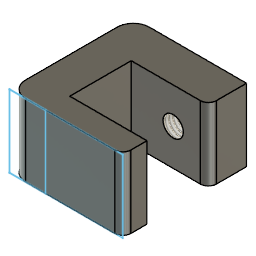
deck2plateClamp_I1 (Autodesk Fusion 360 design; units mm, degrees)
part number: 2026-05-03-05-26-52-082
Autodesk Fusion 360 part; units mm, degrees
sketch "Sketch1" plane through (0, 0, 0) normal (0, 1, 0) x (1, 0, 0)
  line L0 (-6.9583, -4.2531) -> (7.1417, -4.2531)
  line L1 (7.1417, -4.2531) -> (7.1417, 4.7469)
  line L2 (7.1417, 4.7469) -> (-6.9583, 4.7469)
  line L3 (-6.9583, 4.7469) -> (-6.9583, -4.2531)
  line L4 (-6.9583, -4.2531) -> (-2.4583, -4.2531)
  line L5 (-2.4583, -4.2531) -> (-2.4583, 4.7469)
  line L6 (-2.4583, 4.7469) -> (-6.9583, 4.7469)
  line L7 (-6.9583, 4.7469) -> (-6.9583, -4.2531)
  dimension "d4" = 14.1
  dimension "d5" = 9
  dimension "d7" = 4.5
  dimension "d8" = 9
  constraint horizontal L0
  constraint vertical L1
  constraint horizontal L2
  constraint vertical L3
  constraint horizontal L4
  constraint vertical L5
  constraint horizontal L6
  constraint vertical L7
  measures "d4" distance of L0.start L0.end
  measures "d5" distance of L0.start L2.end
  measures "d7" distance of L0.start L4.end
  measures "d8" distance of L0.start L2.end
extrude "Extrude1" add sketch "Sketch1" along normal blind 15.4 contours L0 L2 L3 L4 L5 L6 L7
extrude "Extrude2" add sketch "Sketch1" along normal blind 3 contours L0 L1 L2 L5
sketch "Sketch2" plane through (-2.4583, 0, 0) normal (1, 0, 0) x (0, 1, 0)
  line L0 (3, 4.2531) -> (3, -4.7469)
  line L1 (3, -4.7469) -> (15.4, -4.7469)
  line L2 (15.4, -4.7469) -> (15.4, 4.2531)
  line L3 (15.4, 4.2531) -> (3, 4.2531)
  line L4 (3, -0.2469) -> (10.4, -0.2469)
  line L5 (15.4, 4.2531) -> (10.6439, 4.2531)
  line L6 (10.6439, 4.2531) -> (10.6439, -4.7469)
  line L7 (10.6439, -4.7469) -> (15.4, -4.7469)
  line L8 (15.4, -4.7469) -> (15.4, 4.2531)
  dimension "d16" = 7.4
  constraint midpoint L0 L4.start
  constraint perpendicular L0 L4
  constraint horizontal L5
  constraint vertical L6
  constraint horizontal L7
  constraint vertical L8
  constraint coincident L1 L6.end
  constraint coincident L2.end L3.start
  measures "d16" distance of L4.start L4.end
extrude "Extrude3" add sketch "Sketch2" along normal blind 9.6 contours L1 L2 L3 L5 L6 L7 L8
hole "Hole1" at (2.7613, 10.6439, -0.1995) direction (0, 1, 0) diameter 2.529 end through all
thread "Thread1" "ISO Metric profile 3.0 M3x0.5 M3x0.5 6H" thread offset 0 thread depth 7.4
fillet "Fillet1" radius 2 1 edges at (-6.9583, 15.4, -0.2469)
fillet "Fillet2" radius 2 1 edges at (-6.9583, 0, -0.2469)
fillet "Fillet3" radius 1 1 edges at (7.1417, 10.6439, -0.2469)
fillet "Fillet4" radius 1 1 edges at (7.1417, 0, -0.2469)
equation "clamp_w = 14.1 mm"
equation "clamp_l = 9 mm"
equation "clamp_bot_thickness = 3 mm"
equation "d4 = clamp_w"
equation "d5 = clamp_l"
equation "clamp_mid_w = 4.5 mm"
equation "d7 = clamp_mid_w"
equation "d8 = clamp_l"
equation "clamp_mid_thickness = wp_gap + clamp_bot_thickness + clamp_top_thickness"
equation "d10 = clamp_mid_thickness"
equation "d12 = clamp_bot_thickness"
equation "clamp_top_thickness = 5 mm"
equation "wp_gap = 7.4 mm"
equation "d16 = wp_gap"
equation "top_clamp_depth = clamp_w - clamp_mid_w"
equation "d18 = top_clamp_depth"
